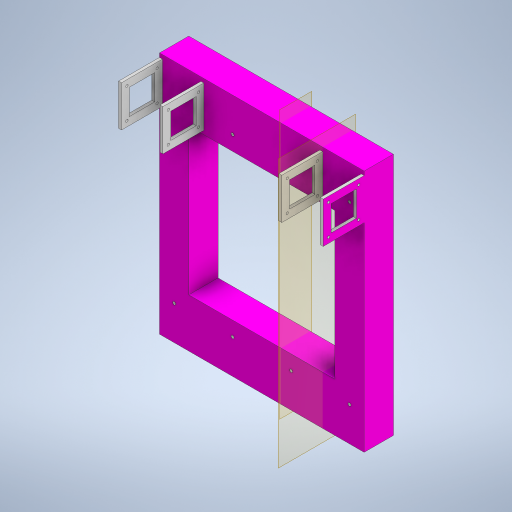
# Autodesk Inventor part: ОСНОВА
Saved by Autodesk Inventor 2024.2 (Build 282272000, 272)
## iProperties
Created: 2025-11-18
Part Number: ОСНОВА
Material: Типовые
Document SubType Name: Modeling
Designer: Zakhar
Density: 1 g/cm^3
Appearance: По умолчанию
Author: Zakhar
Autodesk Inventor part; units mm, degrees
ref_plane "XZ Plane" through (0, 0, 0) normal (0, 1, 0) x (-1, 0, 0)
ref_plane "XY Plane" through (0, 0, 0) normal (0, 0, 1) x (1, 0, 0)
sketch "Эскиз1" plane through (0, 0, 0) normal (0, 0, 1) x (1, 0, 0)
  line L0 (75, -75) -> (-75, -75)
  line L1 (-75, -75) -> (-75, 75)
  line L2 (-75, 75) -> (75, 75)
  line L3 (75, 75) -> (75, -75)
  line L4 (105, -125) -> (-105, -125)
  line L5 (-105, -125) -> (-105, 125)
  line L6 (-105, 125) -> (105, 125)
  line L7 (105, 125) -> (105, -125)
  point P0 (0, 0)
  point P1 (-75, 0)
  point P2 (0, -125)
  point P3 (-105, 0)
  dimension "d0" = 210
  dimension "d1" = 250
  dimension "d3" = 150
  dimension "d4" = 150
  dimension "d5" = 125
  dimension "d6" = 105
  dimension "d7" = 75
  dimension "d8" = 75
  constraints: 16 end point, 4 parallel, 3 midpoint, 2 horizontal, 2 perpendicular
  measures "d0" distance of L4.start L4.end
  measures "d1" distance of L6.end L4.start
  measures "d3" distance of L1.end L2.end
  measures "d4" distance of L0.end L1.end
  measures "d5" distance of point (0, 0) point (0, -125)
  measures "d6" distance of point (-105, 0) point (0, 0)
  measures "d7" distance from line of L0 point (0, 0)
  measures "d8" distance of point (-75, 0) point (0, 0)
extrude "Выдавливание1" add sketch "Эскиз1" along normal blind 30
sketch "Эскиз2" plane through (0, 0, 30) normal (0, 0, 1) x (1, 0, 0)
  circle A0 centre (90, -90) radius 1.5
  line L0 (75, 75) -> (75, -75) projected
  line L1 (-105, 125) -> (-105, -125) projected
  line L2 (90, -90) -> (84.6408, -90) construction
  line L3 (84.6408, -90) -> (90, -90)
  line L4 (90, -90) -> (90, -87.0291) construction
  circle A1 centre (-90, -90) radius 1.5
  circle A2 centre (90, 90) radius 1.5
  circle A3 centre (-90, 90) radius 1.5
  circle A4 centre (30, 90) radius 1.5
  circle A5 centre (30, -90) radius 1.5
  circle A6 centre (-30, 90) radius 1.5
  circle A7 centre (-30, -90) radius 1.5
  point P0 (0, 0)
  point P1 (75, 0)
  dimension "d11" = 3
  dimension "d12" = 90
  dimension "d13" = 195
  dimension "d16" = 180
  dimension "d19" = 180
  dimension "d24" = 60
  constraints: 8 centre point, 6 end point, 3 horizontal, 2 vertical, 1 collinear, 1 midpoint, 14 other
  measures "d11" diameter of A0
  measures "d12" vertical distance of point (75, 0) L2.start
  measures "d13" distance from line of L1 L2.start
  measures "d16" distance of L2.start A1.centre
  measures "d19" distance of L2.start A2.centre
  measures "d24" distance of A2.centre A4.centre
extrude "Выдавливание2" cut sketch "Эскиз2" against normal through all
ref_plane "РабПлоскость4" through (19.7, 0, 0) normal (1, 0, 0) x (0, 1, 0)
sketch "Эскиз7" plane through (105, 0, 0) normal (1, 0, 0) x (0, 1, 0)
  line L0 (79, 30) -> (121, 30)
  line L1 (121, 30) -> (121, 38)
  line L2 (121, 38) -> (79, 38)
  line L3 (79, 38) -> (79, 30)
  line L4 (121, 30) -> (113, 30)
  line L5 (113, 30) -> (113, 72)
  line L6 (113, 72) -> (121, 72)
  line L7 (121, 72) -> (121, 30)
  line L8 (121, 72) -> (79, 72)
  line L9 (79, 72) -> (79, 64)
  line L10 (79, 64) -> (121, 64)
  line L11 (121, 64) -> (121, 72)
  line L12 (79, 72) -> (87, 72)
  line L13 (87, 72) -> (87, 30)
  line L14 (87, 30) -> (79, 30)
  line L15 (79, 30) -> (79, 72)
  line L16 (75, 30) -> (125, 30) construction
  circle A0 centre (84.5, 66.5) radius 1.25
  circle A1 centre (115.5, 66.5) radius 1.25
  circle A2 centre (115.5, 35.5) radius 1.25
  circle A3 centre (84.5, 35.5) radius 1.25
  point P0 (0, 0)
  point P1 (117, 72)
  point P2 (113, 38)
  point P3 (87, 38)
  point P4 (87, 64)
  point P5 (113, 64)
  dimension "d80" = 42
  dimension "d81" = 42
  dimension "d82" = 8
  dimension "d83" = 8
  dimension "d84" = 4
  dimension "d85" = 8
  dimension "d86" = 8
  dimension "d87" = 2.5
  dimension "d88" = 5.5
  dimension "d89" = 5.5
  dimension "d90" = 2.5
  dimension "d91" = 2.5
  dimension "d92" = 2.5
  dimension "d93" = 5.5
  dimension "d94" = 5.5
  dimension "d95" = 5.5
  dimension "d96" = 5.5
  dimension "d97" = 5.5
  dimension "d98" = 5.5
  constraints: 34 end point, 8 parallel, 4 centre point, 4 horizontal, 4 perpendicular, 2 collinear, 1 midpoint, 1 point on line
  measures "d80" distance of L0.start L0.end
  measures "d81" distance of L14.end L8.end
  measures "d82" distance between parallel lines of L6 L10
  measures "d83" distance between parallel lines of L0 L2
  measures "d84" distance from line of L3 L16.start
  measures "d85" distance between parallel lines of L15 L13
  measures "d86" distance between parallel lines of L7 L5
  measures "d87" diameter of A0
  measures "d88" distance from line of L12 A0.centre
  measures "d89" distance from line of L15 A0.centre
  measures "d90" diameter of A1
  measures "d91" diameter of A2
  measures "d92" diameter of A3
  measures "d93" distance from line of L14 A3.centre
  measures "d94" distance from line of L15 A3.centre
  measures "d95" distance from line of L1 A2.centre
  measures "d96" distance from line of L4 A2.centre
  measures "d97" distance from line of L7 A1.centre
  measures "d98" vertical distance of point (117, 72) A1.centre
extrude "Выдавливание5" add sketch "Эскиз7" against normal blind 3 contours L3 L2 L13 L0 | L13 L2 L5 L0 | L15 L10 L13 L2 | L5 L2 L1 L0 | L9 L8 L13 L10 | L5 L10 L7 L2 | L13 L8 L5 L10 | L5 L6 L7 L10
mirror "Зеркальное отражение3" about plane through (0, 0, 0) normal (1, 0, 0) of "Выдавливание5"
ref_plane "РабПлоскость5" through (62.5, -125, 0) normal (1, 0, 0) x (0, 0, -1)
sketch "Эскиз8" plane through (62.5, -125, 0) normal (1, 0, 0) x (0, 0, -1)
  line L0 (-30, 204) -> (-30, 250) construction
  line L1 (-30, 204) -> (-38, 204)
  line L2 (-38, 204) -> (-38, 246)
  line L3 (-38, 246) -> (-30, 246)
  line L4 (-30, 246) -> (-30, 204)
  line L5 (-30, 246) -> (-72, 246)
  line L6 (-72, 246) -> (-72, 238)
  line L7 (-72, 238) -> (-30, 238)
  line L8 (-30, 238) -> (-30, 246)
  line L9 (-72, 246) -> (-64, 246)
  line L10 (-64, 246) -> (-64, 204)
  line L11 (-64, 204) -> (-72, 204)
  line L12 (-72, 204) -> (-72, 246)
  line L13 (-72, 204) -> (-30, 204)
  line L14 (-30, 204) -> (-30, 212)
  line L15 (-30, 212) -> (-72, 212)
  line L16 (-72, 212) -> (-72, 204)
  circle A0 centre (-66.5, 209.5) radius 1.25
  circle A1 centre (-66.5, 240.5) radius 1.25
  circle A2 centre (-35.5, 240.5) radius 1.25
  circle A3 centre (-35.5, 209.5) radius 1.25
  point P0 (0, 125)
  point P1 (-34, 204)
  point P2 (-30, 242)
  point P3 (-38, 238)
  point P4 (-38, 212)
  point P5 (-64, 212)
  point P6 (-64, 238)
  dimension "d102" = 8
  dimension "d103" = 8
  dimension "d104" = 8
  dimension "d105" = 8
  dimension "d106" = 42
  dimension "d107" = 4
  dimension "d108" = 42
  dimension "d109" = 5.5
  dimension "d110" = 5.5
  dimension "d111" = 5.5
  dimension "d112" = 5.5
  dimension "d113" = 5.5
  dimension "d114" = 5.5
  dimension "d115" = 5.5
  dimension "d116" = 5.5
  dimension "d117" = 2.5
  dimension "d118" = 2.5
  dimension "d119" = 2.5
  dimension "d120" = 2.5
  constraints: 34 end point, 8 parallel, 4 centre point, 4 horizontal, 4 perpendicular, 2 midpoint, 1 collinear, 1 point on line
  measures "d102" distance between parallel lines of L0 L2
  measures "d103" distance between parallel lines of L5 L7
  measures "d104" distance between parallel lines of L13 L15
  measures "d105" distance between parallel lines of L12 L10
  measures "d106" distance of L3.end L5.end
  measures "d107" distance from line of L0.end L5
  measures "d108" distance of L11.end L5.end
  measures "d109" distance from line of L12 A1.centre
  measures "d110" distance from line of L9 A1.centre
  measures "d111" distance from line of L16 A0.centre
  measures "d112" distance from line of L11 A0.centre
  measures "d113" vertical distance of point (-34, 204) A3.centre
  measures "d114" distance from line of L14 A3.centre
  measures "d115" distance from line of L5 A2.centre
  measures "d116" horizontal distance of point (-30, 242) A2.centre
  measures "d117" diameter of A2
  measures "d118" diameter of A3
  measures "d119" diameter of A0
  measures "d120" diameter of A1
extrude "Выдавливание6" add sketch "Эскиз8" against normal blind 3 contours L1 L2 L15 L4 | L13 L10 L15 L2 | L15 L2 L7 L4 | L11 L12 L15 L10 | L7 L2 L3 L4 | L7 L10 L5 L2 | L15 L12 L7 L10 | L7 L6 L5 L10
mirror "Зеркальное отражение4" about plane through (0, 0, 0) normal (1, 0, 0) of "Выдавливание6"
